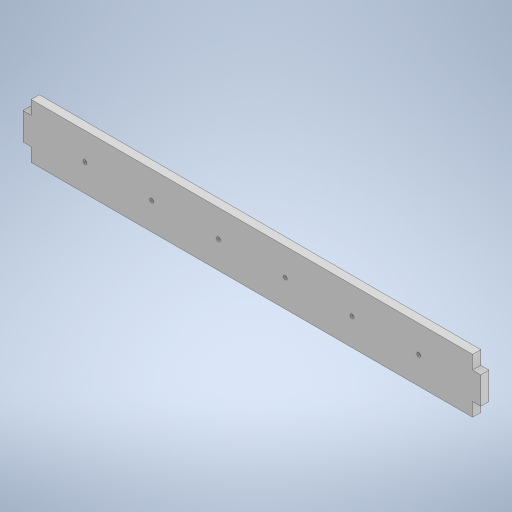
# Autodesk Inventor part: pi_holder
Saved by Autodesk Inventor 2023 (Build 270158000, 158)
## iProperties
Created: 2022-07-08
Part Number: pi_holder
Material: Generic
Document SubType Name: Modeling
Designer: Zayed
Density: 1 g/cm^3
Appearance: Default
Author: Zayed
Autodesk Inventor part; units mm, degrees
ref_plane "YZ Plane" through (0, 0, 0) normal (1, 0, 0) x (0, 1, 0)
ref_plane "XZ Plane" through (0, 0, 0) normal (0, 1, 0) x (-1, 0, 0)
ref_plane "XY Plane" through (0, 0, 0) normal (0, 0, 1) x (1, 0, 0)
sketch "Sketch1" plane through (0, 0, 0) normal (0, 0, 1) x (1, 0, 0)
  line L0 (0, 0) -> (162, 0)
  line L1 (162, 0) -> (162, 20)
  line L2 (-162, -20) -> (162, -20)
  line L3 (162, -20) -> (162, 20)
  line L4 (162, 20) -> (-162, 20)
  line L5 (-162, 20) -> (-162, -20)
  line L6 (-162, -20) -> (162, 20) construction
  line L7 (162, -20) -> (-162, 20) construction
  line L8 (0, 0) -> (24.5, 0)
  line L9 (0, 0) -> (-24.5, 0)
  line L10 (162, 0) -> (165, 0)
  line L11 (162, 0) -> (162, 10)
  line L12 (168, -10) -> (162, -10)
  line L13 (162, -10) -> (162, 10)
  line L14 (162, 10) -> (168, 10)
  line L15 (168, 10) -> (168, -10)
  line L16 (168, -10) -> (162, 10) construction
  line L17 (162, -10) -> (168, 10) construction
  circle A0 centre (24.5, 0) radius 1.35
  circle A1 centre (-24.5, 0) radius 1.35
  line L18 (-162, 0) -> (-165, 0)
  line L19 (-162, 0) -> (-162, 10)
  line L20 (-168, -10) -> (-162, -10)
  line L21 (-162, -10) -> (-162, 10)
  line L22 (-162, 10) -> (-168, 10)
  line L23 (-168, 10) -> (-168, -10)
  line L24 (-168, -10) -> (-162, 10) construction
  line L25 (-162, -10) -> (-168, 10) construction
  line L26 (-24.5, 0) -> (-73.5, 0)
  line L27 (24.5, 0) -> (73.5, 0)
  circle A2 centre (-73.5, 0) radius 1.35
  circle A3 centre (73.5, 0) radius 1.35
  line L28 (73.5, 0) -> (122.5, 0)
  line L29 (-73.5, 0) -> (-122.5, 0)
  circle A4 centre (-122.5, 0) radius 1.35
  circle A5 centre (122.5, 0) radius 1.35
  dimension "d13" = 162
  dimension "d14" = 20
  dimension "d15" = 24.5
  dimension "d16" = 24.5
  dimension "d17" = 3
  dimension "d18" = 10
  dimension "d19" = 2.7
  dimension "d20" = 2.7
  dimension "d21" = 3
  dimension "d22" = 10
  dimension "d25" = 49
  dimension "d26" = 49
  dimension "d27" = 2.7
  dimension "d28" = 2.7
  dimension "d29" = 49
  dimension "d30" = 49
  dimension "d31" = 2.7
  dimension "d32" = 2.7
  constraints: 60 end point, 9 horizontal, 7 midpoint, 6 centre point, 6 coincident, 6 parallel, 5 point on line, 3 perpendicular, 1 vertical
  measures "d13" distance of L0.start L0.end
  measures "d14" distance of L0.end L1.end
  measures "d15" distance of L0.start L8.end
  measures "d16" distance of L0.start L9.end
  measures "d17" distance of L0.end L10.end
  measures "d18" distance of L0.end L11.end
  measures "d19" diameter of A0
  measures "d20" diameter of A1
  measures "d21" distance of L18.start L18.end
  measures "d22" distance of L18.start L19.end
  measures "d25" distance of L26.start L26.end
  measures "d26" distance of L27.start L27.end
  measures "d27" diameter of A2
  measures "d28" diameter of A3
  measures "d29" distance of L28.start L28.end
  measures "d30" distance of L29.start L29.end
  measures "d31" diameter of A4
  measures "d32" diameter of A5
extrude "Extrusion2" add sketch "Sketch1" along normal blind 6
body "Solid2"
